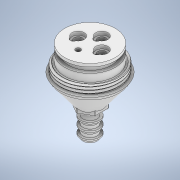
# Autodesk Inventor part: Bottom-V3
Saved by Autodesk Inventor 2021 (Build 250183000, 183)
## iProperties
Created: 2021-08-11
Part Number: Bottom-V3
Material: ABS Plastic
Document SubType Name: Modeling
Designer: incep
Density: 1.06 g/cm^3
Appearance: Smooth - White
Author: incep
## iProperties of the stored document _3DPrint.ipt
Created: 2021-08-11
Part Number: _3DPrint
Material: Generic
Document SubType Name: Modeling
Designer: incep
Density: 1 g/cm^3
Appearance: Default
Author: incep
Autodesk Inventor part; units mm, degrees
ref_plane "YZ Plane" through (0, 0, 0) normal (1, 0, 0) x (0, 1, 0)
ref_plane "XZ Plane" through (0, 0, 0) normal (0, 1, 0) x (-1, 0, 0)
ref_plane "XY Plane" through (0, 0, 0) normal (0, 0, 1) x (1, 0, 0)
sketch "Bottom Sketch - 3/8inTube" plane through (0, 0, 0) normal (0, 0, 1) x (1, 0, 0)
  line L0 (-17, 0) -> (17, 0) construction
  line L1 (17, 0) -> (17, -11) construction
  line L2 (17, -11) -> (-17, -11) construction
  line L3 (-17, -11) -> (-17, 0) construction
  line L4 (-14.5, 0) -> (14.5, 0) construction
  line L5 (14.5, 0) -> (14.5, -8) construction
  line L6 (14.5, -8) -> (-14.5, -8) construction
  line L7 (-14.5, -8) -> (-14.5, 0) construction
  line L8 (17, -11) -> (17, -5.8)
  line L9 (17, -5.8) -> (14.5, -5.8)
  line L10 (14.5, -5.8) -> (14.5, -2)
  line L11 (14.5, -2) -> (17, -2)
  line L12 (17, -2) -> (17, 0)
  line L13 (17, -11) -> (19.65, -11)
  line L14 (-6.5, 0) -> (6.5, 0) construction
  line L15 (6.5, 0) -> (6.5, -37) construction
  line L16 (6.5, -37) -> (-6.5, -37) construction
  line L17 (-6.5, -37) -> (-6.5, 0) construction
  line L18 (19.65, -11) -> (19.65, -17)
  line L19 (17, 0) -> (0, 0)
  line L20 (-4.7625, -37) -> (4.7625, -37) construction
  line L21 (4.7625, -55) -> (-4.7625, -55) construction
  line L22 (-4.7625, -55) -> (-4.7625, -37) construction
  line L23 (6.5, -37) -> (4.7625, -37)
  line L24 (4.7625, -55) -> (3.0125, -55)
  line L25 (3.0125, -55) -> (3.0125, -33.5523)
  line L26 (0, 0) -> (0, -18)
  line L27 (0, -18) -> (14.6768, -18)
  line L28 (14.6768, -18) -> (3.0125, -33.5523)
  line L29 (-2.006, -37) -> (2.006, -37) construction
  line L30 (2.006, -37) -> (2.006, -55) construction
  line L31 (2.006, -55) -> (-2.006, -55) construction
  line L32 (-2.006, -55) -> (-2.006, -37) construction
  line L33 (4.7625, -52) -> (6.2625, -52) construction
  line L34 (6.2625, -52) -> (6.2625, -55) construction
  line L35 (6.2625, -55) -> (4.7625, -55) construction
  line L36 (4.7625, -55) -> (4.7625, -52) construction
  line L37 (4.7625, -47) -> (6.2625, -47) construction
  line L38 (6.2625, -47) -> (6.2625, -50) construction
  line L39 (6.2625, -50) -> (4.7625, -50) construction
  line L40 (4.7625, -50) -> (4.7625, -47) construction
  line L41 (4.7625, -42) -> (6.2625, -42) construction
  line L42 (6.2625, -42) -> (6.2625, -45) construction
  line L43 (6.2625, -45) -> (4.7625, -45) construction
  line L44 (4.7625, -45) -> (4.7625, -42) construction
  line L45 (4.7625, -55) -> (6.2625, -53)
  line L46 (6.2625, -52) -> (6.2625, -53)
  line L47 (6.2625, -52) -> (4.7625, -52)
  line L48 (4.7625, -50) -> (6.2625, -48)
  line L49 (6.2625, -48) -> (6.2625, -47)
  line L50 (6.2625, -47) -> (4.7625, -47)
  line L51 (4.7625, -45) -> (6.2625, -43)
  line L52 (6.2625, -43) -> (6.2625, -42)
  line L53 (6.2625, -42) -> (4.7625, -42)
  line L54 (4.7625, -37) -> (4.7625, -42)
  line L55 (4.7625, -37) -> (4.7625, -47) construction
  line L56 (4.7625, -50) -> (4.7625, -52) construction
  line L57 (4.7625, -45) -> (4.7625, -47)
  line L58 (4.7625, -50) -> (4.7625, -52)
  line L59 (-22.5, 0) -> (22.5, 0) construction
  line L60 (22.5, 0) -> (22.5, -17) construction
  line L61 (22.5, -17) -> (-22.5, -17) construction
  line L62 (-22.5, -17) -> (-22.5, 0) construction
  line L63 (-21.5, 0) -> (21.5, 0) construction
  line L64 (21.5, 0) -> (21.5, -17) construction
  line L65 (21.5, -17) -> (-21.5, -17) construction
  line L66 (-21.5, -17) -> (-21.5, 0) construction
  line L67 (22.5, 0) -> (21.7206, -13.2491) construction
  line L68 (19.694, -19.408) -> (6.5, -37) construction
  arc A0 (19.694, -19.408) -> (21.0266, -17) centre (11.694, -13.408) ccw
  line L69 (19.65, -17) -> (21.0266, -17)
  line L70 (6.5, -37) -> (6.5, -37)
  line L71 (6.5, -37) -> (6.5, -37)
  line L72 (6.5, -37) -> (19.694, -19.408)
  point P0 (0, -8)
  point P1 (0, -37)
  point P2 (0, -37)
  point P3 (0, -37)
  point P4 (0, -55)
  point P5 (0, -55)
  dimension "d0" = 11
  dimension "d1" = 8
  dimension "d2" = 34
  dimension "d3" = 29
  dimension "d4" = 2
  dimension "d5" = 3.8
  dimension "d6" = 37
  dimension "d7" = 13
  dimension "d8" = 9.525
  dimension "d9" = 18
  dimension "d10" = 1.75
  dimension "d11" = 18
  dimension "d16" = 1.5
  dimension "d18" = 3
  dimension "d19" = 1.5
  dimension "d20" = 3
  dimension "d21" = 2
  dimension "d22" = 1.5
  dimension "d23" = 3
  dimension "d24" = 2
  dimension "d25" = 17
  dimension "d26" = 1
  dimension "d27" = 1
  dimension "d28" = 1
  dimension "d29" = 17
  dimension "d30" = 45
  dimension "d31" = 17
  dimension "d32" = 43
  dimension "d33" = 10
  dimension "d87" = 19.65
  dimension "d112" = 6.5
  dimension "d117" = 0
  dimension "d118" = 3.0125
  constraints: 146 end point, 22 parallel, 17 perpendicular, 14 coincident, 14 collinear, 13 horizontal, 13 point on line, 11 midpoint, 2 point on circle, 2 tangent, 2 vertical, 2 vertical alignment, 1 centre point
  measures "d0" distance of L1.start L8.start
  measures "d1" distance of L5.start L5.end
  measures "d2" distance of L8.start L2.end
  measures "d3" distance of L5.end L6.end
  measures "d4" distance of L11.end L1.start
  measures "d5" distance of L9.end L10.end
  measures "d6" distance of L15.end L15.start
  measures "d7" distance of L15.end L17.start
  measures "d8" distance of L24.start L22.start
  measures "d9" distance of L20.end L24.start
  measures "d10" distance of L24.start L25.start
  measures "d11" distance of L19.end L26.end
  measures "d16" distance of L34.end L24.start
  measures "d18" distance of L33.end L34.end
  measures "d19" distance of L38.end L39.end
  measures "d20" distance of L37.end L38.end
  measures "d21" distance of L33.start L39.end
  measures "d22" distance of L42.end L43.end
  measures "d23" distance of L41.end L42.end
  measures "d24" distance of L37.start L43.end
  measures "d25" vertical distance of L18.end point (0, 0)
  measures "d26" distance of L33.end L45.end
  measures "d27" distance of L48.end L37.end
  measures "d28" distance of L51.end L41.end
  measures "d29" distance of L61.end L59.start
  measures "d30" distance of L60.end L61.end
  measures "d31" distance of L65.end L63.start
  measures "d32" distance of L63.start L63.end
  measures "d33" radius of A0
  measures "d87" horizontal distance of L18.start point (0, 0)
  measures "d112" distance from line of L71 point (0, 0)
  measures "d117" distance of L70.end L71.end
  measures "d118" horizontal distance of L25.start point (0, 0)
revolve "Bottom" add sketch "Bottom Sketch - 3/8inTube" angle 360 about axis through (0, 0, 0) along (0, -1, 0)
sketch "Sketch2" plane through (0, 0, 0) normal (0, 1, 0) x (1, 0, 0)
  circle A0 centre (8, 0) radius 2.725
  circle A1 centre (0, 8) radius 2.725
  circle A2 centre (-8, 0) radius 2.725
  circle A3 centre (0, -8) radius 1.65
  point P0 (0, 0)
  point P1 (0, 0)
  point P2 (0, 0)
  dimension "d37" = 8
  dimension "d38" = 5.45
  dimension "d41" = 180
  dimension "d43" = 8
  dimension "d44" = 3.3
  constraints: 4 centre point, 1 coincident, 6 other
  measures "d37" distance of A0.centre point (0, 0)
  measures "d38" diameter of A0
  measures "d43" distance of A3.centre point (0, 0)
  measures "d44" diameter of A3
extrude "Extrusion1" cut sketch "Sketch2" against normal blind 19
sketch "Sketch3" plane through (0, 0, 0) normal (0, 1, 0) x (1, 0, 0)
  circle A0 centre (8, 0) radius 4.075
  circle A1 centre (0, 8) radius 4.075
  circle A2 centre (-8, 0) radius 4.075
  point P0 (0, 0)
  point P1 (0, 0)
  point P2 (0, 0)
  dimension "d47" = 8.15
  dimension "d49" = 8
  dimension "d52" = 180
  constraints: 3 centre point, 1 coincident, 1 horizontal alignment, 6 other
  measures "d47" diameter of A0
  measures "d49" distance of A0.centre point (0, 0)
extrude "Extrusion2" cut sketch "Sketch3" against normal blind 2.36
sketch "Sketch4" plane through (0, 0, 0) normal (0, 1, 0) x (1, 0, 0)
  circle A0 centre (0, 8) radius 2.725 projected
  circle A1 centre (0, 4.662) radius 2
  circle A2 centre (8, 0) radius 2.725 projected
  circle A3 centre (8, -3.2496) radius 2
  circle A4 centre (-8, 0) radius 2.725 projected
  circle A5 centre (-8, -3.2496) radius 2
  point P0 (0, 0)
  dimension "d56" = 4
  dimension "d57" = 4
  dimension "d58" = 4
  constraints: 3 centre point
  measures "d56" diameter of A1
  measures "d57" diameter of A3
  measures "d58" diameter of A5
extrude "Extrusion3" cut sketch "Sketch4" against normal blind 19 contours A1 A0 | A0 A1 | A3 A2 | A2 A3 | A5 A4 | A4 A5 picked at (0.3506, 5.7392) picked at (-0.5374, 4.5206) picked at (8.3617, -2.2316) picked at (8.5627, -3.4363) picked at (-7.6383, -2.2316) picked at (-7.4373, -3.4363)
thread "Thread6" size "M42x2" class "6g" standard "ANSI Metric M Profile" length 6
sketch "Sketch9" plane through (0, -17, 0) normal (-1, 0, 0) x (0, 0, 1)
  line L0 (19.65, 0) -> (19.65, 6)
  line L1 (19.65, 6) -> (18.1671, 6)
  line L2 (18.1671, 6) -> (18.1671, 0)
  line L3 (18.1671, 0) -> (19.65, 0)
  line L4 (0, -1.2) -> (0, 7.2) projected
  constraints: 8 end point
revolve "Revolution5" cut sketch "Sketch9" angle 360 about axis through (0, -17, 0) along (0, 1, 0)
sketch "Sketch10" plane through (0, -17, 0) normal (-1, 0, 0) x (0, 0, 1)
  line L0 (19.65, 0) -> (19.65, 6)
  line L1 (19.65, 6) -> (18.1671, 6)
  line L2 (18.1671, 6) -> (18.1671, 0)
  line L3 (18.1671, 0) -> (19.65, 0)
  line L4 (0, -1.2) -> (0, 7.2) projected
  constraints: 8 end point
revolve "Revolution6" add sketch "Sketch10" angle 360 about axis through (0, -17, 0) along (0, 1, 0) separate body
sketch "Sketch8" plane through (0, -17, 0) normal (1, 0, 0) x (0, 1, 0)
  line L0 (-1.1668, -18.2684) -> (-1.0001, -18.2684) construction
  line L1 (0.1666, -19.549) -> (-0.0001, -19.8692) construction
  line L2 (-2.0001, -19.8692) -> (-2.1668, -19.549) construction
  line L3 (-0.8334, -18.2684) -> (-1.0001, -17.9482) construction
  line L4 (-1.0001, -17.9482) -> (-1.1668, -18.2684) construction
  line L5 (-2.0001, -19.8692) -> (-1.8334, -19.549) construction
  line L6 (-0.8334, -18.2684) -> (-0.1668, -19.549)
  line L7 (-2.1668, -19.549) -> (-1.8334, -19.549) construction
  arc A0 (-2.1668, -19.549) -> (-2.0001, -19.6502) centre (-2.0001, -19.4623) ccw construction
  line L8 (0.1666, -19.549) -> (-0.1668, -19.549) construction
  line L9 (-2.0001, -19.8692) -> (-2.0001, -19.549) construction
  line L10 (-0.0001, -19.8692) -> (-0.0001, -19.549) construction
  line L11 (-1.0001, -17.9482) -> (-1.0001, -18.1672) construction
  line L12 (-2.0001, -19.6502) -> (-0.0001, -19.6502)
  arc A1 (-2.0001, -19.6502) -> (-1.8334, -19.549) centre (-2.0001, -19.4623) ccw
  line L13 (-0.1668, -19.549) -> (-0.0001, -19.8692) construction
  line L14 (-1.8334, -19.549) -> (-1.1668, -18.2684)
  line L15 (-0.0001, -0.0002) -> (-0.0001, 0.0177)
  line L16 (-0.0001, 0.0177) -> (-0.0001, -0.0002)
  line L17 (-0.0001, -0.0002) -> (0.0334, -0.0002)
  arc A2 (-0.1668, -19.549) -> (-0.0001, -19.6502) centre (-0.0001, -19.4623) ccw
  arc A3 (-0.0001, -19.6502) -> (0.1666, -19.549) centre (-0.0001, -19.4623) ccw construction
  arc A4 (-1.0001, -18.1672) -> (-1.1668, -18.2684) centre (-1.0001, -18.3551) ccw
  arc A5 (-0.8334, -18.2684) -> (-1.0001, -18.1672) centre (-1.0001, -18.3551) ccw
  line L18 (-1.0001, -18.1672) -> (-1.0001, -18.2684) construction
  line L19 (-1.0001, -18.2684) -> (-0.8334, -18.2684) construction
  dimension "d92" = 55
  dimension "d93" = 0.3202
  dimension "d94" = 0.3202
  dimension "Sketch8_ThreadOffset" = 0
  dimension "Sketch8_MajorRadius" = 19.65
  dimension "d97" = 2
  dimension "Sketch8_MinorRadius" = 18.1671
  constraints: 40 end point, 12 point on circle, 10 parallel, 8 tangent, 6 centre point, 6 collinear, 2 midpoint, 2 point on line, 1 horizontal, 1 perpendicular, 3 other
  measures "d92" angle of L6 L14
  measures "d93" distance of L3.end L0.end
  measures "d94" distance of L1.end L10.end
  measures "Sketch8_ThreadOffset" distance between parallel lines of L15 L10
  measures "Sketch8_MajorRadius" distance from line of L12 L15.start
  measures "d97" distance from line of L1.end L9
  measures "Sketch8_MinorRadius" distance edge to line of A5 L17
coil "Coil2" sketch "Sketch8" operation cut axis through (0, -17, 0) along (0, 1, 0) pitch 2.002 turns 4.995005 hand right bodies 2
sketch "Sketch11" plane through (0, -37, 0) normal (0, -1, 0) x (1, 0, 0)
  line L0 (8, -4.6188) -> (0, -9.2376)
  line L1 (0, -9.2376) -> (-8, -4.6188)
  line L2 (-8, -4.6188) -> (-8, 4.6188)
  line L3 (-8, 4.6188) -> (0, 9.2376)
  line L4 (0, 9.2376) -> (8, 4.6188)
  line L5 (8, 4.6188) -> (8, -4.6188)
  circle A0 centre (0, 0) radius 6
  dimension "d113" = 8
  dimension "d119" = 12
  constraints: 12 end point, 2 coincident, 1 centre point, 13 other
  measures "d113" distance from line of L5 point (0, 0)
  measures "d119" diameter of A0
extrude "Extrusion6" add sketch "Sketch11" against normal blind 5 bodies 1
fillet "Fillet1" radius 0.75 12 edges at (-8, -35.1749, 4.6188) (-8, -37, 0) (-8, -35.1749, -4.6188) (-4, -37, -6.9282) (0, -35.1749, -9.2376) (4, -37, -6.9282) (8, -35.1749, -4.6188) (8, -35.1749, 4.6188) (8, -37, 0) (4, -37, 6.9282) (0, -35.1749, 9.2376) (-4, -37, 6.9282)
equation "\"d70\" = 0.1875"
equation "\"Sketch5_Pitch\" = 1.5"
equation "\"d72\" = 60deg"
equation "\"d99\" = 55deg"
equation "\"Sketch8_Pitch\" = 2"
body "Solid2"
body "Solid4"
